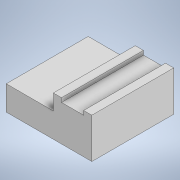
# Autodesk Inventor part: Rackhalter
Saved by Autodesk Inventor 2021 (Build 250183000, 183)
## iProperties
Created: 2025-04-11
Part Number: Rackhalter
Material: Generic
Document SubType Name: Modeling
Designer: Lukas
Density: 1 g/cm^3
Appearance: Default
Author: Lukas
Autodesk Inventor part; units mm, degrees
ref_plane "YZ Plane" through (0, 0, 0) normal (1, 0, 0) x (0, 1, 0)
ref_plane "XZ Plane" through (0, 0, 0) normal (0, 1, 0) x (-1, 0, 0)
ref_plane "XY Plane" through (0, 0, 0) normal (0, 0, 1) x (1, 0, 0)
sketch "Sketch1" plane through (0, 0, 0) normal (0, 0, 1) x (1, 0, 0)
  line L0 (0, 0) -> (20.9, 0)
  line L1 (20.9, 0) -> (20.9, 9.8)
  line L2 (20.9, 9.8) -> (18.9, 9.8)
  line L3 (18.9, 9.8) -> (18.9, 8.8)
  line L4 (18.9, 8.8) -> (13.5, 8.8)
  line L5 (13.5, 8.8) -> (13.5, 9.8)
  line L6 (13.5, 9.8) -> (11.5, 9.8)
  line L7 (11.5, 9.8) -> (11.5, 6)
  line L8 (11.5, 6) -> (0, 6)
  line L9 (0, 6) -> (0, 0)
  dimension "d0" = 13.5
  dimension "d1" = 8.8
  dimension "d2" = 5.4
  dimension "d3" = 1
  dimension "d4" = 2
  dimension "d5" = 6
  constraints: 20 end point, 6 perpendicular, 2 horizontal, 2 point on line, 1 collinear, 1 parallel
  measures "d0" distance between parallel lines of L9 L5
  measures "d1" distance between parallel lines of L0 L4
  measures "d2" distance of L3.end L4.end
  measures "d3" distance of L2.end L3.end
  measures "d4" distance of L1.end L2.end
  measures "d5" distance of L8.end L0.start
extrude "Extrusion1" add sketch "Sketch1" along normal blind 20
sketch "Sketch2" plane through (0, 0, 0) normal (-1, 0, 0) x (0, 0, 1)
  circle A0 centre (3, 3) radius 1.4
  circle A1 centre (17, 3) radius 1.4
  line L0 (0, 0) -> (20, 0) projected
  point P0 (10, 0)
  dimension "d8" = 3
  dimension "d9" = 14
  dimension "d10" = 2.8
  dimension "d11" = 7
  constraints: 2 centre point, 1 equal radius, 1 horizontal alignment, 1 midpoint
  measures "d8" distance from line of L0 A0.centre
  measures "d9" distance of A1.centre A0.centre
  measures "d10" diameter of A0
  measures "d11" horizontal distance of A0.centre point (10, 0)
extrude "Extrusion2" cut sketch "Sketch2" against normal blind 10
equation "\"d11\" = 0.5 * d9"
body "Solid1"
